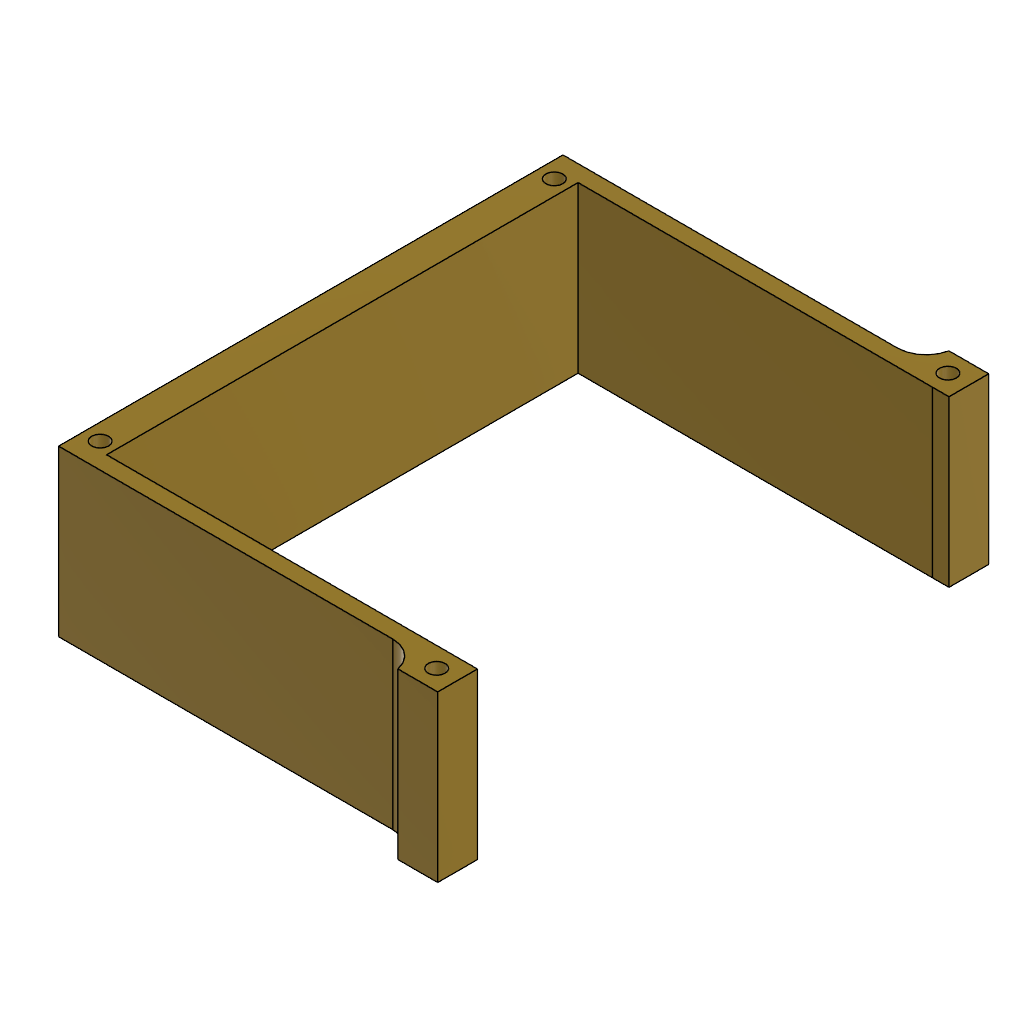
only+ups+box+plate (Autodesk Fusion 360 design; units mm, degrees)
part number: 2026-08-26-12-24-20-880
Autodesk Fusion 360 part; units mm, degrees
sketch "Sketch1" plane through (0, 0, 0) normal (0, 0, 1) x (1, 0, 0)
  line L0 (27.37, 56.6) -> (117.87, 56.6)
  line L1 (117.87, 56.6) -> (117.87, -56.6)
  line L2 (117.87, -56.6) -> (27.37, -56.6)
  line L3 (27.37, -56.6) -> (27.37, 56.6)
  line L4 (27.37, 56.6) -> (117.87, -56.6) construction
  line L5 (117.87, 56.6) -> (27.37, -56.6) construction
  line L6 (21.37, -84) -> (-39.63, -84)
  line L7 (-39.63, -84) -> (-39.63, 84)
  line L8 (-39.63, 84) -> (21.37, 84)
  line L9 (21.37, 84) -> (21.37, -84)
  line L10 (21.37, -84) -> (-39.63, 84) construction
  line L11 (-39.63, -84) -> (21.37, 84) construction
  line L12 (0, 183.4733) -> (0, -140)
  line L13 (22.37, -85) -> (-40.63, -85)
  line L14 (-40.63, -85) -> (-40.63, 85)
  line L15 (-40.63, 85) -> (22.37, 85)
  line L16 (22.37, 85) -> (22.37, -85)
  line L17 (24.87, -87.5) -> (-43.13, -87.5)
  line L18 (-43.13, -87.5) -> (-43.13, 87.5)
  line L19 (-43.13, 87.5) -> (24.87, 87.5)
  line L20 (24.87, 87.5) -> (24.87, -87.5)
  line L21 (118.37, -57.1) -> (26.87, -57.1)
  line L22 (26.87, -57.1) -> (26.87, 57.1)
  line L23 (26.87, 57.1) -> (118.37, 57.1)
  line L24 (118.37, 57.1) -> (118.37, -57.1)
  line L25 (120.37, -59.1) -> (24.87, -59.1)
  line L26 (24.87, -59.1) -> (24.87, 59.1)
  line L27 (24.87, 59.1) -> (120.37, 59.1)
  line L28 (120.37, 59.1) -> (120.37, -59.1)
  line L29 (120.37, 59.1) -> (135.37, 59.1) construction
  line L30 (135.37, 59.1) -> (135.37, -59.1) construction
  line L31 (135.37, 59.1) -> (135.37, 74.1) construction
  line L32 (32.52, 57.1) -> (112.72, 57.1)
  line L33 (112.72, 57.1) -> (112.72, -57.1)
  line L34 (112.72, -57.1) -> (32.52, -57.1)
  line L35 (32.52, -57.1) -> (32.52, 57.1)
  line L36 (32.52, 57.1) -> (112.72, -57.1) construction
  line L37 (112.72, 57.1) -> (32.52, -57.1) construction
  line L38 (118.37, -57.1) -> (135.37, -57.1114)
  line L39 (118.37, 57.1) -> (135.37, 57.0972)
  line L40 (120.37, -59.1) -> (112.72, -59.1)
  line L41 (112.72, -59.1) -> (112.72, -66.75)
  line L42 (112.72, -66.75) -> (120.37, -66.75)
  line L43 (120.37, -66.75) -> (120.37, -59.1)
  line L44 (120.37, 59.1) -> (112.72, 59.1)
  line L45 (112.72, 59.1) -> (112.72, 66.75)
  line L46 (112.72, 66.75) -> (120.37, 66.75)
  line L47 (120.37, 66.75) -> (120.37, 59.1)
  line L48 (14.87, 85) -> (14.87, 87.5)
  line L49 (-33.13, 85) -> (-33.13, 87.5)
  line L50 (22.37, 85) -> (24.87, 87.5)
  line L51 (-40.63, 85) -> (-43.13, 87.5)
  line L52 (-40.63, -85) -> (-43.13, -87.5)
  line L53 (-40.63, -85) -> (-43.13, -87.5)
  line L54 (22.37, -85) -> (24.87, -87.5)
  line L55 (14.87, -85) -> (14.87, -87.5)
  line L56 (-33.13, -85) -> (-33.13, -87.5)
  line L57 (136.62, 105) -> (-73.38, 105)
  line L58 (-73.38, 105) -> (-73.38, -105)
  line L59 (-73.38, -105) -> (136.62, -105)
  line L60 (136.62, -105) -> (136.62, 105)
  line L61 (31.62, 105) -> (31.62, -105)
  line L62 (136.62, 105) -> (-73.38, -105) construction
  line L63 (136.62, -105) -> (-73.38, 105) construction
  line L64 (136.62, 105) -> (136.62, 75) construction
  line L65 (136.62, 75) -> (122.4779, 60.8579) construction
  line L66 (136.62, 75) -> (156.62, 75) construction
  line L67 (122.4779, 60.8579) -> (122.4779, 90.8579) construction
  line L68 (122.4779, 90.8579) -> (92.4779, 90.8579) construction
  line L69 (92.4779, 90.8579) -> (106.62, 105) construction
  line L70 (106.62, 105) -> (136.62, 105) construction
  line L71 (129.5489, 67.9289) -> (129.5489, 97.9289) construction
  line L72 (129.5489, 97.9289) -> (99.5489, 97.9289) construction
  line L73 (122.4779, 66.9579) -> (136.62, 81.1) construction
  line L74 (122.4779, 66.9579) -> (141.8419, 66.9579) construction
  circle A0 centre (129.5489, 74.0289) radius 1.55
  circle A1 centre (129.5489, 74.0289) radius 2.8
  line L75 (122.37, 59.1) -> (122.37, 66.75)
  line L76 (122.37, 66.75) -> (120.37, 66.75)
  line L77 (120.37, -66.75) -> (122.37, -66.75)
  line L78 (122.37, -66.75) -> (122.37, -59.1)
  line L79 (122.37, -59.1) -> (120.37, -59.1)
  line L80 (122.37, 59.1) -> (122.3697, 57.0993)
  line L81 (122.3697, 57.0993) -> (120.37, 57.0997)
  line L82 (120.37, 57.0997) -> (120.37, 59.1)
  line L83 (122.37, -59.1) -> (122.3713, -57.1027)
  line L84 (-9.13, 0) -> (-43.13, 0) construction
  line L85 (-43.13, -30) -> (-40.13, -30)
  line L86 (-40, -30) -> (-40, -70)
  line L87 (-40, -70) -> (-43.13, -70)
  line L88 (-43.13, 30) -> (-40.13, 30)
  line L89 (-40.13, 30) -> (-40.13, 70)
  line L90 (-40.13, 70) -> (-43.13, 70)
  line L91 (24.87, 30) -> (21.87, 30)
  line L92 (21.87, 30) -> (21.87, 70)
  line L93 (21.87, 70) -> (25.2263, 70.1588)
  line L94 (24.87, -30) -> (21.87, -30)
  line L95 (21.87, -30) -> (21.87, -70)
  line L96 (21.87, -70) -> (24.87, -70)
  line L97 (-40.13, -30) -> (-40, -70)
  point P0 (72.62, 0)
  point P1 (-9.13, 0)
  point P2 (0, -102.5)
  point P3 (0, 102.5)
  point P4 (72.62, 0)
  dimension "d90" = 38.25
  dimension "d91" = 38.25
  dimension "d92" = 111.75
  dimension "d93" = 68
  dimension "d94" = 175
  dimension "d95" = 10
  dimension "d96" = 17.5
  dimension "d97" = 21
  dimension "d98" = -1
  dimension "d100" = 210
  dimension "d101" = 9.13
  dimension "d102" = 7.65
  dimension "d103" = 113.2
  dimension "d104" = 95.5
  dimension "d105" = -0.5
  dimension "d106" = 72.62
  dimension "d107" = 57.1
  dimension "d108" = 32.52
  dimension "d109" = 47.9
  dimension "d110" = 82.9
  dimension "d111" = 45.4
  dimension "d112" = 159.6
  dimension "d113" = 240.5733
  dimension "d119" = 30
  dimension "d120" = 135
  dimension "d121" = 20
  dimension "d122" = 30
  dimension "d123" = 45
  dimension "d124" = 45
  dimension "d125" = 6.1
  dimension "d126" = 3.1
  dimension "d129" = 5.6
  dimension "d140" = 2
  dimension "d141" = 2
  dimension "d142" = 114.1993
  dimension "d143" = 109.3219
  dimension "d173" = 3
  dimension "d174" = 40
  dimension "d175" = 3
  dimension "d176" = 40
  dimension "d177" = 3
  dimension "d178" = 40
  dimension "d179" = 3
  dimension "d180" = 40
  dimension "d181" = 30
  dimension "d182" = 30
  dimension "d183" = 30
  dimension "d184" = 30
  dimension "d185" = 70
  dimension "d186" = 30.87
  dimension "d187" = 70.1588
  constraint horizontal L0
  constraint perpendicular L0 L1
  constraint parallel L0 L2
  constraint parallel L1 L3
  constraint coincident L4 P4
  constraint coincident L5 P4
  constraint horizontal L6
  constraint perpendicular L6 L7
  constraint parallel L6 L8
  constraint parallel L7 L9
  constraint coincident L10 P1
  constraint coincident L11 P1
  constraint perpendicular L6 L12
  constraint coincident origin L12
  constraint coincident L12 P2
  constraint coincident L12 P3
  constraint perpendicular L28 L29
  constraint perpendicular L25 L30
  constraint perpendicular L29 L31
  constraint horizontal L32
  constraint perpendicular L32 L33
  constraint parallel L32 L34
  constraint parallel L33 L35
  constraint coincident L36 P4
  constraint coincident L37 P4
  constraint coincident L30 L39.end
  constraint equal L38 L39
  constraint horizontal L40
  constraint vertical L41
  constraint horizontal L42
  constraint vertical L43
  constraint horizontal L44
  constraint vertical L45
  constraint horizontal L46
  constraint vertical L47
  constraint collinear L33 L41
  constraint coincident L15 L48.start
  constraint coincident L19 L48.end
  constraint perpendicular L19 L48
  constraint coincident L15 L49.start
  constraint coincident L19 L49.end
  constraint perpendicular L19 L49
  constraint coincident L13 L55.start
  constraint coincident L17 L55.end
  constraint perpendicular L17 L55
  constraint coincident L13 L56.start
  constraint coincident L17 L56.end
  constraint perpendicular L17 L56
  constraint horizontal L57
  constraint vertical L58
  constraint horizontal L59
  constraint vertical L60
  constraint equal L57 L58
  constraint midpoint L57 L61.start
  constraint midpoint L59 L61.end
  constraint coincident L20 L26.end
  constraint coincident L21 L34.end
  constraint coincident L23 L32.end
  constraint equal L29 L31
  constraint equal L26 L30
  constraint perpendicular L57 L64
  constraint horizontal L66
  constraint coincident L62 L67.end
  constraint parallel L31 L67
  constraint perpendicular L67 L68
  constraint coincident L57 L69.end
  constraint midpoint L65 L71.start
  constraint coincident L62 L71.end
  constraint parallel L64 L71
  constraint midpoint L69 L72.end
  constraint horizontal L74
  constraint coincident L67 L73.start
  constraint coincident L60 L73.end
  constraint midpoint L73 A0.centre
  constraint concentric A0 A1
  constraint perpendicular L46 L75
  constraint perpendicular L47 L76
  constraint perpendicular L43 L77
  constraint perpendicular L40 L78
  constraint perpendicular L43 L79
  constraint coincident L39 L80.end
  constraint perpendicular L39 L80
  constraint coincident L28 L81.end
  constraint coincident L39 L81.end
  constraint coincident L38 L83.end
  constraint perpendicular L38 L83
  constraint equal L65 L66
  constraint coincident P1 L84.start
  constraint midpoint L18 L84.end
  constraint coincident L18 L85.start
  constraint perpendicular L14 L85
  constraint perpendicular L85 L86
  constraint coincident L18 L87.end
  constraint perpendicular L18 L87
  constraint coincident L18 L88.start
  constraint perpendicular L14 L88
  constraint perpendicular L88 L89
  constraint coincident L18 L90.end
  constraint perpendicular L18 L90
  constraint coincident L26 L91.start
  constraint perpendicular L26 L91
  constraint perpendicular L91 L92
  constraint coincident L26 L94.start
  constraint perpendicular L20 L94
  constraint perpendicular L94 L95
  constraint coincident L20 L96.end
  constraint perpendicular L20 L96
  measures "d90" distance of L46.end L57
  measures "d91" distance of L42.end L59
  measures "d92" distance of L26 L60
  measures "d93" distance of L17.start L17.end
  measures "d94" distance of L17.end L18.end
  measures "d95" distance of L17.end L56.end
  measures "d96" distance of L19 L57
  measures "d97" distance of L8 L57
  measures "d100" distance of L57.start L57.end
  measures "d101" distance of origin P1
  measures "d102" distance of L25.start L42.end
  measures "d103" distance of L0.end L1.end
  measures "d104" distance of L25.start L25.end
  measures "d106" distance of origin P4
  measures "d107" distance of origin L34
  measures "d108" distance of origin L35
  measures "d109" distance of L34 L59
  measures "d110" distance of L12.end L34
  measures "d111" distance of P2 L34
  measures "d112" distance of P3 L34
  measures "d113" distance of L12.start L34
  measures "d119" distance of L57.start L64.end
  measures "d120" angle of L65 L66
  measures "d121" distance of L64.end L65.end
  measures "d122" distance of L67.end L68.end
  measures "d123" angle of L68 L69
  measures "d124" angle of L73 L74
  measures "d125" distance of L65.end L73.start
  measures "d126" diameter of A0
  measures "d129" diameter of A1
  measures "d140" distance of L27.end L75.start
  measures "d141" distance of L42.end L77.end
  measures "d142" distance of L34 L80.end
  measures "d143" distance of L35 L74.end
  measures "d173" distance of L85.start L85.end
  measures "d174" distance of L86.start L86.end
  measures "d175" distance of L88.start L88.end
  measures "d176" distance of L88.end L89.end
  measures "d177" distance of L91.start L91.end
  measures "d178" distance of L91.end L92.end
  measures "d179" distance of L94.start L94.end
  measures "d180" distance of L94.end L95.end
  measures "d181" vertical distance of origin L94.end
  measures "d182" vertical distance of P1 L85.end
  measures "d183" vertical distance of origin L91.end
  measures "d184" distance of L84.end L88.start
  measures "d185" distance of L84 L87
  measures "d186" distance of P1 L86
  measures "d187" distance of L84 L93.end
extrude "Extrude1" add sketch "Sketch1" against normal blind 5 contours L0 L2 L3 L21 L22 L23 L61 | L0 L2 L3 L61 | L0 L23 L35 L61 | L0 L2 L35 L61 | L0 L23 L32 L33 L35 | L0 L2 L33 L35 | L23 L27 L28 L32 L39 L44 L61 L82 | L20 L21 L22 L23 L25 L26 L27 L61 | L2 L21 L35 L61 | L0 L1 L2 L21 L23 L24 L33 | L0 L1 L2 L33 | L2 L21 L33 L34 L35 | L21 L25 L28 L34 L38 L40 L61 | L16 L20 L26 L91 L93 | L24 L28 L38 L39 | L16 L20 L26 L91 L94 | L16 L20 L50 L93 | L16 L20 L26 L94 L96 | L16 L91 L92 L93 | L6 L8 L9 L12 L13 L15 L16 L91 L92 L93 L94 L95 L96 | L15 L19 L48 L50 | L12 L15 L19 L48 | L12 L15 L19 L49 | L16 L20 L54 L96 | L16 L94 L95 L96 | L6 L7 L8 L12 L13 L14 L15 L85 L87 L88 L89 L90 L97 | L15 L19 L49 L51 | L13 L17 L54 L55 | L12 L13 L17 L56 | L12 L13 L17 L55 | L6 L7 L8 L12 | L6 L8 L9 L12 | L14 L18 L51 L90 | L13 L17 L52 L53 L56 | L14 L18 L88 L90 | L14 L18 L52 L53 L87 | L14 L88 L89 L90 | L14 L18 L85 L88 | L14 L18 L85 L87 | L14 L85 L87 L97 makes body 1
extrude "Extrude2" cut sketch "Sketch1" against normal blind 3 contours L0 L23 L32 L33 L35 | L0 L2 L33 L35 | L2 L21 L33 L34 L35 | L16 L91 L92 L93 | L6 L8 L9 L12 L13 L15 L16 L91 L92 L93 L94 L95 L96 | L16 L94 L95 L96 | L6 L7 L8 L12 L13 L14 L15 L85 L87 L88 L89 L90 L97 | L6 L7 L8 L12 | L6 L8 L9 L12 | L14 L88 L89 L90 | L14 L85 L87 L97 bodies 1
extrude "Extrude4" cut sketch "Sketch1" against normal blind 1.5 contours L0 L1 L2 L21 L23 L24 L33 | L0 L1 L2 L33 | L25 L27 L28 L38 L39 L41 L42 L45 L46 L57 L59 L60 L61 L75 L76 L77 L78 L80 L81 L83 | L24 L28 L38 L39 | A1 bodies 1
extrude "Extrude5" add sketch "Sketch1" along normal blind 40 contours L0 L2 L3 L21 L22 L23 L61 | L0 L2 L3 L61 | L0 L23 L35 L61 | L0 L2 L35 L61 | L23 L27 L28 L32 L39 L44 L61 L82 | L20 L21 L22 L23 L25 L26 L27 L61 | L2 L21 L35 L61 | L21 L25 L28 L34 L38 L40 L61 | L27 L44 L45 L46 L47 | L25 L40 L41 L42 L43 bodies 1
extrude "Extrude6" cut sketch "Sketch1" against normal up to surface (3 mm away) contours L0 L1 L2 L21 L23 L24 L33 | L0 L1 L2 L33 | L24 L28 L38 L39 bodies 1
extrude "Extrude9" add sketch "Sketch1" against normal blind 4 contours L0 L2 L3 L21 L22 L23 L61 | L0 L2 L3 L61 | L0 L23 L35 L61 | L0 L2 L35 L61 | L0 L23 L32 L33 L35 | L0 L2 L33 L35 | L23 L27 L28 L32 L39 L44 L61 L82 | L20 L21 L22 L23 L25 L26 L27 L61 | L2 L21 L35 L61 | L0 L1 L2 L21 L23 L24 L33 | L0 L1 L2 L33 | L2 L21 L33 L34 L35 | L25 L27 L28 L38 L39 L41 L42 L45 L46 L57 L59 L60 L61 L75 L76 L77 L78 L80 L81 L83 | L12 L19 L20 L27 L57 L61 | L21 L25 L28 L34 L38 L40 L61 | L16 L20 L26 L91 L93 | L27 L44 L45 L46 L47 | L12 L17 L20 L25 L59 L61 | L24 L28 L38 L39 | L16 L20 L26 L91 L94 | L16 L20 L50 L93 | L28 L39 L47 L75 L76 L80 L81 L82 | L12 L17 L18 L19 L57 L58 L59 | L25 L40 L41 L42 L43 | L16 L20 L26 L94 L96 | L16 L91 L92 L93 | L6 L8 L9 L12 L13 L15 L16 L91 L92 L93 L94 L95 L96 | L15 L19 L48 L50 | L12 L15 L19 L48 | L12 L15 L19 L49 | L43 L77 L78 L79 | L28 L38 L79 L83 | L16 L20 L54 L96 | L16 L94 L95 L96 | L6 L7 L8 L12 L13 L14 L15 L85 L87 L88 L89 L90 L97 | L15 L19 L49 L51 | L13 L17 L54 L55 | L12 L13 L17 L56 | L12 L13 L17 L55 | L6 L7 L8 L12 | L6 L8 L9 L12 | L14 L18 L51 L90 | L13 L17 L52 L53 L56 | L14 L18 L88 L90 | L14 L18 L52 L53 L87 | L14 L88 L89 L90 | L14 L18 L85 L88 | L14 L18 L85 L87 | L14 L85 L87 L97 | A0 | A1 bodies 1
ref_plane "WorkPlane3" through (136.62, 105, 0) normal (0.707107, -0.707107, 0) x (0.707107, 0.707107, 0)
fillet "Fillet2" radius 2 4 edges at (136.62, 105, -2) (-73.38, 105, -2) (-73.38, -105, -2) (136.62, -105, -2) on bodies 1
sketch "Sketch2" plane through (0, 0, 0) normal (0, 0, 1) x (1, 0, 0)
  line L0 (31.62, -0.363) -> (31.62, 105.8348)
  line L1 (31.62, -0.363) -> (31.62, -104.355)
  circle A0 centre (31.62, -75) radius 1.6
  circle A1 centre (31.62, 75) radius 1.6
  line L2 (134.62, 105) -> (-71.38, 105)
  line L3 (-71.38, -105) -> (134.62, -105)
  line L4 (31.62, -105) -> (31.62, 105)
  line L5 (136.62, -110.9828) -> (136.62, 124.515) construction
  point P0 (31.62, -0.363)
  dimension "d81" = 0.363
  dimension "d82" = 3.2
  dimension "d83" = 3.2
  dimension "d114" = 210
  dimension "d115" = 105
  dimension "d117" = 75.363
  dimension "d118" = 74.637
  dimension "d144" = 0.645
  dimension "d145" = 210.1897
  dimension "d146" = 5.9828
  dimension "d147" = 235.4977
  constraint coincident P0 L0.start
  constraint vertical L0
  constraint parallel L0 L1
  constraint coincident L1 A0.centre
  constraint coincident L0 A1.centre
  constraint midpoint L3 L4.start
  constraint midpoint L2 L4.end
  constraint perpendicular L3 L5
  measures "d81" vertical distance of origin L0.start
  measures "d82" diameter of A0
  measures "d83" diameter of A1
  measures "d115" distance of L0 L5
  measures "d117" distance of P0 A1.centre
  measures "d118" distance of P0 A0.centre
  measures "d144" distance of L1.end L3
  measures "d145" vertical distance of L0.end L1.end
  measures "d146" distance of L3 L5.start
  measures "d147" vertical distance of L5.start L5.end
extrude "Extrude10" cut sketch "Sketch2" against normal up to surface (4 mm away) bodies 1
extrude "Extrude11" cut sketch "Sketch1" against normal blind 6 contours A0 bodies 1
extrude "Extrude12" cut sketch "Sketch1" against normal blind 3 from surface at -1.5 contours A1 bodies 1
ref_plane "WorkPlane1" through (31.62, 0, -2) normal (0, 1, 0) x (1, 0, 0)
ref_plane "WorkPlane2" through (31.62, 0, -2) normal (1, 0, 0) x (0, -1, 0)
mirror "Mirror1" about plane through (136.62, 105, 0) normal (0.707107, -0.707107, 0) of "Extrude11", "Extrude12"
mirror "Mirror2" about plane through (31.62, 0, -2) normal (1, 0, 0) of "Extrude11", "Extrude12", "Mirror1"
mirror "Mirror3" about plane through (31.62, 0, -2) normal (0, 1, 0) of "Extrude11", "Extrude12", "Mirror1", "Mirror2"
extrude "Extrude13" add sketch "Sketch1" along normal up to surface (40 mm away) contours L28 L39 L47 L75 L76 L80 L81 L82 | L43 L77 L78 L79 | L28 L38 L79 L83 bodies 1
sketch "Sketch3" plane through (0, 0, 40) normal (0, 0, 1) x (-1, 0, 0)
  line L0 (-112.72, 66.75) -> (-122.37, 66.75)
  line L1 (-122.37, 66.75) -> (-122.37, 59.1)
  line L2 (-122.37, 59.1) -> (-122.3713, 57.1027)
  line L3 (-122.3713, 57.1027) -> (-118.37, 57.1)
  line L4 (-118.37, 57.1) -> (-32.52, 57.1)
  line L5 (-32.52, 57.1) -> (-32.52, -57.1)
  line L6 (-32.52, -57.1) -> (-118.37, -57.1)
  line L7 (-118.37, -57.1) -> (-122.3697, -57.0993)
  line L8 (-122.3697, -57.0993) -> (-122.37, -59.1)
  line L9 (-122.37, -59.1) -> (-122.37, -66.75)
  line L10 (-122.37, -66.75) -> (-112.72, -66.75)
  line L11 (-24.87, -59.1) -> (-24.87, 59.1)
  circle A0 centre (-117.295, -61.925) radius 2.05
  circle A1 centre (-117.295, -61.925) radius 1.6
  circle A2 centre (-28.8623, -55.0092) radius 2.05
  circle A3 centre (-28.8623, -55.0092) radius 1.6
  circle A4 centre (-28.87, 55.0168) radius 2.05
  circle A5 centre (-28.87, 55.0168) radius 1.6
  circle A6 centre (-117.295, 61.925) radius 2.05
  circle A7 centre (-117.295, 61.925) radius 1.6
  line L12 (-112.72, 59.1) -> (-112.72, 66.75)
  line L13 (-112.72, -66.75) -> (-112.72, -59.1)
  line L14 (-112.72, -59.1) -> (-24.87, -59.1)
  line L15 (-24.87, 59.1) -> (-112.72, 59.1)
  dimension "d150" = 4.1
  dimension "d151" = 3.2
  dimension "d152" = 4.1
  dimension "d153" = 3.2
  dimension "d154" = 4.1
  dimension "d155" = 3.2
  dimension "d156" = 4.1
  dimension "d157" = 3.2
  dimension "d158" = 5.075
  dimension "d159" = 5.075
  dimension "d160" = 4.825
  dimension "d161" = 4.825
  dimension "d162" = 4
  dimension "d163" = 110.026
  dimension "d164" = 5.716
  dimension "d165" = 5.716
  constraint concentric A0 A1
  constraint concentric A2 A3
  constraint concentric A4 A5
  constraint concentric A6 A7
  measures "d150" diameter of A0
  measures "d151" diameter of A1
  measures "d152" diameter of A2
  measures "d153" diameter of A3
  measures "d154" diameter of A4
  measures "d155" diameter of A5
  measures "d156" diameter of A6
  measures "d157" diameter of A7
  measures "d158" distance of L1 A6.centre
  measures "d159" distance of L9 A0.centre
  measures "d160" distance of L10 A0.centre
  measures "d161" distance of L0 A6.centre
  measures "d162" distance of L11 A4.centre
  measures "d163" vertical distance of A2.centre A4.centre
  measures "d164" distance of L11.start A2.centre
  measures "d165" distance of L11.end A4.centre
extrude "Extrude14" cut sketch "Sketch3" against normal blind 8 contours A1 | A3 | A5 | A7 bodies 1
extrude "Extrude15" cut sketch "Sketch3" against normal blind 4.5 contours A0 | A2 | A4 | A6 bodies 1
extrude "Extrude16" cut 1 faces at (88.5367, 19.7, -5) along direction (0, 0, 1) blind 1 on bodies 1 bodies 1
split "Split1" by plane through (0, 0, 0) normal (0, 0, 1) bodies 1 makes body 2 at (24.87, 19.7, 26.6667)
extrude "Extrude17" cut sketch "Sketch1" against normal up to surface (4 mm away) contours L16 L20 L26 L91 L93 | L16 L20 L26 L94 L96 | L16 L91 L92 L93 | L16 L94 L95 L96 | L14 L18 L88 L90 | L14 L88 L89 L90 | L14 L18 L85 L87 | L14 L85 L87 L97 bodies 1
sketch "Sketch4" plane through (0, 0, -4) normal (0, 0, -1) x (1, 0, 0)
  arc A0 (136.62, 103) -> (134.62, 105) centre (134.62, 103) ccw
  line L0 (134.62, 105) -> (-71.38, 105)
  arc A1 (-71.38, 105) -> (-73.38, 103) centre (-71.38, 103) ccw
  line L1 (-73.38, 103) -> (-73.38, -103)
  arc A2 (-73.38, -103) -> (-71.38, -105) centre (-71.38, -103) ccw
  line L2 (-71.38, -105) -> (134.62, -105)
  arc A3 (134.62, -105) -> (136.62, -103) centre (134.62, -103) ccw
  line L3 (136.62, -103) -> (136.62, 103)
  circle A4 centre (31.62, -75) radius 1.6
  circle A5 centre (31.62, 75) radius 1.6
  circle A6 centre (129.5489, -74.0289) radius 2.8
  circle A7 centre (105.6489, -97.9289) radius 2.8
  circle A8 centre (-66.3089, -74.0289) radius 2.8
  circle A9 centre (-42.4089, -97.9289) radius 2.8
  circle A10 centre (129.5489, 74.0289) radius 2.8
  circle A11 centre (105.6489, 97.9289) radius 2.8
  circle A12 centre (-42.4089, 97.9289) radius 2.8
  circle A13 centre (-66.3089, 74.0289) radius 2.8
  line L4 (-40, 70) -> (-40.13, 30)
  line L5 (-40.13, 30) -> (-43.13, 30)
  line L6 (-43.13, 30) -> (-43.13, 70)
  line L7 (-43.13, 70) -> (-40, 70)
  line L8 (-43.13, -70) -> (-43.13, -30)
  line L9 (-43.13, -30) -> (-40.13, -30)
  line L10 (-40.13, -30) -> (-40.13, -70)
  line L11 (-40.13, -70) -> (-43.13, -70)
  line L12 (21.87, 70) -> (24.87, 70)
  line L13 (24.87, 70) -> (24.87, 30)
  line L14 (24.87, 30) -> (21.87, 30)
  line L15 (21.87, 30) -> (21.87, 70)
  line L16 (21.87, -30) -> (24.87, -30)
  line L17 (24.87, -30) -> (24.87, -70.142)
  line L18 (24.87, -70.142) -> (21.87, -70)
  line L19 (21.87, -70) -> (21.87, -30)
  circle A14 centre (28.87, 55.0168) radius 1.6
  circle A15 centre (28.8623, -55.0092) radius 1.6
  circle A16 centre (117.295, -61.925) radius 1.6
  circle A17 centre (117.295, 61.925) radius 1.6
  circle A18 centre (28.87, 55.0168) radius 1.6
  circle A19 centre (28.87, 55.0168) radius 2.055
  circle A20 centre (117.295, 61.925) radius 1.6
  circle A21 centre (117.295, 61.925) radius 2.05
  circle A22 centre (117.295, -61.925) radius 1.6
  circle A23 centre (117.295, -61.925) radius 2.05
  circle A24 centre (28.8623, -55.0092) radius 1.6
  circle A25 centre (28.8623, -55.0092) radius 2.05
  dimension "d190" = 4.11
  dimension "d191" = 4.1
  dimension "d192" = 4.1
  dimension "d193" = 4.1
  dimension "d194" = 3.2
  constraint concentric A14 A18
  constraint concentric A14 A19
  constraint concentric A17 A20
  constraint concentric A17 A21
  constraint concentric A16 A22
  constraint concentric A22 A23
  constraint concentric A15 A24
  constraint concentric A15 A25
  constraint equal A14 A18
  constraint equal A14 A22
  constraint equal A14 A24
  measures "d190" diameter of A19
  measures "d191" diameter of A21
  measures "d192" diameter of A23
  measures "d193" diameter of A25
  measures "d194" diameter of A20
extrude "Extrude18" cut sketch "Sketch4" against normal blind 11 contours A14 A18 | A15 A24 | A16 A22 | A17 A20 bodies 1 2
extrude "Extrude19" cut sketch "Sketch4" against normal blind 2 contours A19 | A21 | A23 | A25 bodies 1
delete_body "RemoveBody1" bodies 1
extrude "Extrude20" cut sketch "Sketch4" against normal blind 5 from surface at -4 contours A19 | A21 | A23 | A25 bodies 2
extrude "Extrude21" add 1 faces at (54.1533, 59.1, 13.3333) along direction (0, 1, 0) blind 2 on bodies 2 bodies 2
extrude "Extrude22" add 1 faces at (83.4367, -59.1, 26.6667) along direction (0, -1, 0) blind 2 on bodies 2 bodies 2
extrude "Extrude23" cut 1 faces at (122.37, -64.2, 13.3333) along direction (1, 0, 0) up to surface end surface through (122.37, -59.1, 0) normal (1, -0.000671, 0) offset 0 on bodies 2 bodies 2
extrude "Extrude24" add 1 faces at (122.37, 61.65, 26.6667) along direction (1, 0, 0) up to surface end surface through (122.37, 59.1, 0) normal (1, -0.000164, 0) offset 0 on bodies 2 bodies 2
fillet "Fillet3" radius 7 2 edges at (112.72, 61.1, 20) (112.72, -61.1, 20) on bodies 2
equation "d159 = d158"
equation "d161 = d160"
named bodies: "plate", "ups box"
